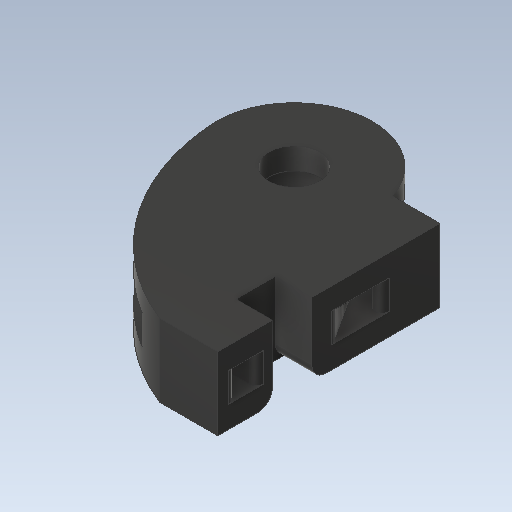
# Autodesk Inventor part: アンテナパーツ
Saved by Autodesk Inventor 2020 (Build 240168000, 168)
## iProperties
Created: 2019-02-02
Part Number: アンテナパーツ
Material: ABS プラスチック
Document SubType Name: Modeling
Designer: ito 017
Density: 1.06 g/cm^3
Appearance: 滑らか - 黒
Author: ito 017
Autodesk Inventor part; units mm, degrees
ref_plane "YZ Plane" through (0, 0, 0) normal (1, 0, 0) x (0, 1, 0)
ref_plane "XZ Plane" through (0, 0, 0) normal (0, 1, 0) x (-1, 0, 0)
ref_plane "XY Plane" through (0, 0, 0) normal (0, 0, 1) x (1, 0, 0)
sketch "スケッチ1" plane through (0, 0, 0) normal (0, 1, 0) x (-1, 0, 0)
  line L0 (0, 0) -> (24, 0)
  line L1 (24, -14.4198) -> (24, -21.5054)
  line L2 (0, -30.5) -> (0, 0)
  line L3 (8, -30.5) -> (8, -33)
  line L4 (8, -33) -> (24, -33)
  line L5 (24, -33) -> (24, -30.5)
  circle A0 centre (16.75, -27.25) radius 5.75
  line L6 (11, -33) -> (11, -13.1635)
  line L7 (0, -7.5) -> (5, -7.5)
  line L8 (5, -7.5) -> (5, -12.9)
  line L9 (5, -12.9) -> (0, -12.9)
  line L10 (0, -12.9) -> (0, -7.5)
  circle A1 centre (16.75, -27.25) radius 10.75
  line L11 (8, -33) -> (8, -33.495)
  line L12 (8, 0) -> (0, 0)
  line L13 (0, 0) -> (0, -6.7624)
  line L14 (0, -6.7624) -> (8, -6.7624)
  line L15 (8, -6.7624) -> (8, 0)
  arc A2 (27.5, -27.25) -> (8, 0) centre (-3.461, -28.8035) ccw
  line L16 (0, -2.5) -> (16.3982, -2.5)
  line L17 (16.3982, -2.5) -> (16.3982, -5)
  line L18 (16.3982, -5) -> (0, -5)
  line L19 (0, -5) -> (0, -2.5)
  line L20 (8, -30.5) -> (0, -18.7731)
  line L21 (12.0066, -30.5) -> (0, -12.9)
  line L22 (0, -15.5617) -> (15.9538, -38.9479)
  line L23 (7, -32.5) -> (0, -32.5)
  line L24 (0, -32.5) -> (0, -40.0084)
  line L25 (0, -40.0084) -> (7, -40.0084)
  line L26 (7, -40.0084) -> (7, -32.5)
  line L27 (0, -19.9979) -> (11.2473, -36.4849)
  arc A3 (25.7114, -33.1877) -> (2.9112, 0) centre (-3.461, -28.8035) ccw
  circle A4 centre (16.75, -27.25) radius 9.25
  line L28 (2.9112, 0) -> (0, 0)
  line L29 (0, -7.5) -> (5, -7.5)
  line L30 (5, -12.9) -> (0, -12.9)
  line L31 (2.9112, 0) -> (0, 0)
  line L32 (0, -7.5) -> (5, -7.5)
  line L33 (5, -12.9) -> (0, -12.9)
  line L34 (0, -30.5) -> (6.503, -30.5)
  line L35 (0, 0) -> (8, 0)
  arc A5 (27.5, -27.25) -> (8, 0) centre (-3.461, -28.8035) ccw
  arc A6 (6.503, -30.5) -> (27.5, -27.25) centre (16.75, -27.25) ccw
  line L36 (8, -33.495) -> (8, -30.5)
  line L37 (24, -30.5) -> (21.4934, -30.5)
  line L38 (12.0066, -30.5) -> (8, -30.5)
  line L39 (24, -30.5) -> (21.4934, -30.5)
  line L40 (12.0066, -30.5) -> (0, -30.5)
  circle A7 centre (16.75, -27.25) radius 5.75
  dimension "d22" = 18.5
  dimension "d0" = 30.5
  dimension "d1" = 24
  dimension "d2" = 2.5
  dimension "d3" = 8
  dimension "d4" = 3
  dimension "d5" = 11.5
  dimension "d6" = 5.75
  dimension "d7" = 7.5
  dimension "d8" = 5
  dimension "d9" = 5.4
  dimension "d10" = 21.5
  dimension "d11" = 8
  dimension "d12" = 31
  dimension "d13" = 2.5
  dimension "d14" = 2.5
  dimension "d17" = 1
  dimension "d18" = 2.5
  dimension "d19" = 1.5
  dimension "d20" = 0
  dimension "d21" = 59
  constraints: 82 end point, 17 parallel, 17 point on circle, 11 point on line, 8 perpendicular, 7 centre point, 7 horizontal, 4 coincident, 4 collinear, 2 tangent, 2 vertical, 1 concentric, 3 other
  measures "d0" distance of L2.start L0.start
  measures "d1" distance of L0.start L0.end
  measures "d2" distance of L4.end L5.end
  measures "d3" distance between parallel lines of L2 L3
  measures "d4" distance between parallel lines of L3 L6
  measures "d5" diameter of A0
  measures "d6" distance from line of L6 A0.centre
  measures "d7" distance between parallel lines of L0 L7
  measures "d8" distance of L7.start L7.end
  measures "d9" distance of L7.end L8.end
  measures "d10" diameter of A1
  measures "d11" distance of L13.end L14.end
  measures "d12" radius of A2
  measures "d13" distance between parallel lines of L16 L18
  measures "d14" distance between parallel lines of L0 L16
  measures "d17" distance between parallel lines of L26 L3
  measures "d18" distance between parallel lines of L27 L22
  measures "d19" distance between parallel lines of L22 L21
  measures "d20" distance of L21.end L9.end
  measures "d21" diameter of A3
extrude "押し出し1" add sketch "スケッチ1" along normal blind 7 contours L0 A3 L15 L16 L2 | L0 L15 A3 | L16 L15 L18 L2 | A2 L16 A3 L15 | A3 L16 L15 | L18 L15 L14 L2 | L16 A3 L18 L15 | A2 L18 A3 L16 | L14 L15 L18 A3 L1 A1 L21 L9 L8 L7 L2 | A2 L1 A3 L18 | A2 A1 A3 L1 | A3 A1 L1 | L21 A1 L22 L2 | A2 A1 A3 | A1 A3 A4 L1 | L1 A4 L6 A1 | L22 A1 L20 L2 | L21 A4 L22 A1 | A1 L6 A4 L21 | A4 A3 L5 L37 A0 L6 | L20 A1 L27 L2 | L22 A4 L38 L20 A1 | A4 L6 L21 | L21 L6 L38 L22 A4 | A1 L22 A4 A3 | L27 A1 L34 L2 | L20 L40 L27 A1 | L22 L38 A4 | L6 A0 L38 | A1 L27 L4 A4 L22 | A0 | A4 L22 L4 | L4 A0 L37 L5 | L27 L40 A1 | L38 A4 L4 L27 L3 | L3 L27 L40 | L38 L6 L22 | L22 L6 L4 A4 L38 | L38 A0 L4 L22 L6 | A1 L11 L4 L27 | A4 L4 L22 | L40 L27 L3 L11 A1 | L27 L4 L3 | L22 L4 L6
sketch "スケッチ3" plane through (0, 7, 0) normal (0, 1, 0) x (1, 0, 0)
  circle A0 centre (-16.75, 27.25) radius 5.75
  arc A1 (-6.503, 30.5) -> (-27.5, 27.25) centre (-16.75, 27.25) ccw projected
  point P0 (0, 0)
  dimension "d25" = 11.5
  constraints: 1 centre point, 1 concentric
  measures "d25" diameter of A0
hole "穴1" at (-16.75, 7, -27.25) direction (0, -1, 0) diameter 11.5 depth 8 tip angle 118
sketch "スケッチ4" plane through (0, 7, 0) normal (0, 1, 0) x (1, 0, 0)
  arc A0 (-12.5853, 35.5094) -> (-7.5065, 27.596) centre (-16.75, 27.25) ccw
  arc A1 (-6.503, 30.5) -> (-27.5, 27.25) centre (-16.75, 27.25) ccw projected
  arc A2 (-27.5, 27.25) -> (-8, 0) centre (3.461, 28.8035) ccw projected
  line L0 (0, 2.5) -> (-9.8946, 2.5)
  line L1 (-14.3641, 5.2979) -> (0, 5.2979)
  line L2 (0, 5.2979) -> (0, 2.5)
  line L3 (-8, 0) -> (0, 0) projected
  line L4 (0, 12.9) -> (0, 30.5) projected
  line L5 (0, 12.9) -> (0, 15.9)
  circle A3 centre (-16.75, 27.25) radius 5.75 projected
  line L6 (0, 20.1285) -> (-12.6428, 39.8275)
  line L7 (-9.8946, 2.5) -> (-12.9439, 2.5)
  arc A4 (-25.9999, 27.2867) -> (-14.3641, 5.2979) centre (3.461, 28.8035) ccw
  arc A5 (-9.8946, 2.5) -> (-2.9112, 0) centre (3.461, 28.8035) ccw
  line L8 (0, 15.9) -> (-12.5853, 35.5094)
  line L9 (-14.2516, 37.7056) -> (-15.4382, 39.5545)
  line L10 (-6.503, 30.5) -> (-6.503, 30.261)
  line L11 (-12.9439, 2.5) -> (0, 2.5)
  line L12 (0, 0) -> (0, 7.5) projected
  dimension "d33" = 18.5
  dimension "d34" = 2.5
  dimension "d36" = 3
  constraints: 20 end point, 9 point on circle, 5 point on line, 3 centre point, 3 parallel, 2 horizontal, 1 coincident, 1 concentric, 1 perpendicular, 1 vertical
  measures "d33" diameter of A0
  measures "d34" distance between parallel lines of L3 L0
  measures "d36" distance of L4.start L5.end
extrude "押し出し2" cut sketch "スケッチ4" against normal blind 4 contours A0 A4 L1 L2 L0 L7 A2 A1 L6 L4 L8 | A4 A0 | L6 A1 L10
sketch "スケッチ5" plane through (0, 7, 0) normal (0, 1, 0) x (1, 0, 0)
  line L0 (-8, 0) -> (0, 0) projected
  line L1 (-8, 0) -> (0, 0)
  line L2 (0, 0) -> (0, 7.5) projected
  line L3 (0, 0) -> (0, 7.5)
  line L4 (0, 7.5) -> (-5, 7.5) projected
  line L5 (0, 7.5) -> (-5, 7.5)
  line L6 (-5, 7.5) -> (-5, 12.9) projected
  line L7 (-5, 7.5) -> (-5, 12.9)
  line L8 (-5, 12.9) -> (0, 12.9)
  line L9 (0, 30.5) -> (-6.503, 30.5) projected
  line L10 (0, 12.9) -> (0, 30.5)
  line L11 (0, 30.5) -> (-6.503, 30.5)
  arc A0 (-6.503, 30.5) -> (-27.5, 27.25) centre (-16.75, 27.25) ccw projected
  arc A1 (-6.503, 30.5) -> (-27.5, 27.25) centre (-16.75, 27.25) ccw
  arc A2 (-27.5, 27.25) -> (-8, 0) centre (3.461, 28.8035) ccw projected
  arc A3 (-27.5, 27.25) -> (-8, 0) centre (3.461, 28.8035) ccw
  constraints: 14 end point, 4 point on circle, 3 collinear, 3 perpendicular, 2 centre point, 1 concentric, 1 horizontal
extrude "押し出し3" add sketch "スケッチ5" along normal blind 3
sketch "スケッチ6" plane through (-16.75, 7, -27.25) normal (0, -1, 0) x (1, 0, 0)
  circle A0 centre (0, 0) radius 3.5
  circle A1 centre (0, 0) radius 5.75 projected
  point P0 (16.75, 27.25)
  dimension "d43" = 7
  constraints: 1 centre point, 1 concentric
  measures "d43" diameter of A0
hole "穴2" at (-16.75, 7, -27.25) direction (0, 1, 0) diameter 7 depth 8 tip angle 118
fillet "フィレット2" radius 1 6 edges at (0, 5, -20.1285) (0, 5, -15.9) (0, 5, -5.2979) (0, 5, -2.5) (-14.3641, 5, -5.2979) (-12.5853, 5, -35.5094)
fillet "フィレット3" radius 2 2 edges at (-2.5, 0, -7.5) (-2.5, 0, -12.9)
